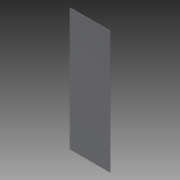
# Autodesk Inventor part: Electronics plate top
Saved by Autodesk Inventor 2015 (Build 190159000, 159)
## iProperties
Created: 2015-01-17
Part Number: Electronics plate top
Material: Generic
Document SubType Name: Modeling
Designer: chapale16
Density: 1 g/cm^3
Appearance: Default
Author: chapale16
Autodesk Inventor part; units mm, degrees
ref_plane "YZ Plane" through (0, 0, 0) normal (1, 0, 0) x (0, 1, 0)
ref_plane "XZ Plane" through (0, 0, 0) normal (0, 1, 0) x (-1, 0, 0)
ref_plane "XY Plane" through (0, 0, 0) normal (0, 0, 1) x (1, 0, 0)
sketch "Sketch2" plane through (0, 0, 0) normal (0, 0, 1) x (1, 0, 0)
  line L0 (0, 0) -> (566.42, 0)
  line L1 (566.42, 0) -> (566.42, -1727.2)
  line L2 (566.42, -1727.2) -> (0, -1727.2)
  line L3 (0, -1727.2) -> (0, 0)
  dimension "d0" = 566.42
  dimension "d1" = 1727.2
  constraints: 8 end point, 2 parallel, 1 horizontal, 1 perpendicular
  measures "d0" distance of L1.end L2.end
  measures "d1" distance of L0.end L1.end
extrude "Extrusion1" add sketch "Sketch2" along normal blind 3.175
sketch "Sketch4" plane through (0, 0, 3.175) normal (0, 0, 1) x (1, 0, 0)
  line L0 (566.42, 0) -> (0, 0) projected
  line L1 (0, 0) -> (0, -1727.2) projected
  line L2 (0, -1727.2) -> (566.42, -1727.2) projected
  line L3 (566.42, -1727.2) -> (566.42, 0) projected
  line L4 (0, -1727.2) -> (566.42, -1727.2) projected
  line L5 (68.58, -1727.2) -> (500.38, -1727.2)
  circle A0 centre (68.58, -1391.92) radius 12.7
  circle A1 centre (500.38, -1391.92) radius 12.7
  circle A2 centre (68.58, -1727.2) radius 12.7
  circle A3 centre (500.38, -1727.2) radius 12.7
  dimension "d6" = 25.4
  dimension "d7" = 25.4
  dimension "d8" = 25.4
  dimension "d9" = 25.4
  constraints: 4 centre point, 2 coincident, 2 end point, 1 horizontal, 1 point on line
  measures "d6" diameter of A0
  measures "d7" diameter of A1
  measures "d8" diameter of A2
  measures "d9" diameter of A3
extrude "Extrusion2" add sketch "Sketch4" along normal blind 3.175 contours A0 | A1
sketch "Sketch6" plane through (0, 0, 3.175) normal (0, 0, 1) x (1, 0, 0)
  circle A0 centre (12.7, -1460.5) radius 3.175 projected
  circle A1 centre (553.72, -1460.5) radius 3.175 projected
  circle A2 centre (553.72, -1460.5) radius 4.7625
  circle A3 centre (12.7, -1460.5) radius 4.7625
  point P0 (0, 0)
  dimension "d16" = 9.525
  dimension "d17" = 9.525
  constraints: 2 centre point, 2 coincident
  measures "d16" diameter of A2
  measures "d17" diameter of A3
extrude "Extrusion4" cut sketch "Sketch6" against normal through all contours A0 | A1 | A2 | A3
sketch "Sketch7" plane through (0, 0, 3.175) normal (0, 0, 1) x (1, 0, 0)
  circle A0 centre (12.7, -1460.5) radius 4.7625 projected
  circle A1 centre (12.7, -1460.5) radius 6.35
  circle A2 centre (553.72, -1460.5) radius 4.7625 projected
  circle A3 centre (553.72, -1460.5) radius 6.35
  point P0 (0, 0)
  dimension "d20" = 12.7
  dimension "d21" = 12.7
  constraints: 2 centre point, 2 coincident
  measures "d20" diameter of A1
  measures "d21" diameter of A3
extrude "Extrusion5" cut sketch "Sketch7" against normal blind 12.7 contours A3
sketch "Sketch9" plane through (0, 0, 3.175) normal (0, 0, 1) x (1, 0, 0)
  circle A0 centre (553.72, -825.5) radius 6.35 projected
  circle A1 centre (12.7, -825.5) radius 6.35 projected
  circle A2 centre (12.7, -825.5) radius 6.35
  circle A3 centre (553.72, -825.5) radius 6.35
  point P0 (0, 0)
  constraints: 2 centre point, 2 coincident, 2 concentric
extrude "Extrusion7" cut sketch "Sketch9" against normal blind 3.175
sketch "Sketch10" plane through (0, 0, 3.175) normal (0, 0, 1) x (1, 0, 0)
  line L0 (566.42, 0) -> (566.42, -1727.2) projected
  line L1 (0, -1732.8892) -> (566.42, -1732.8892)
  line L2 (566.42, -1732.8892) -> (566.42, -1054.0894)
  line L3 (566.42, -1054.0894) -> (0, -1054.0894)
  line L4 (0, -1054.0894) -> (0, -1732.8892)
  point P0 (0, 0)
  constraints: 8 end point, 2 parallel, 1 horizontal, 1 perpendicular, 1 point on line
extrude "Extrusion8" cut sketch "Sketch10" along normal blind 25.4
equation "\"d22\" = d20"
body "Solid1"
